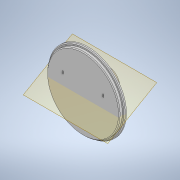
# Autodesk Inventor part: V4Lid
Saved by Autodesk Inventor 2021 (Build 250183000, 183)
## iProperties
Created: 2022-01-21
Part Number: V4Lid
Material: Generic
Document SubType Name: Sheet Metal
Designer: Unit-005
Density: 1 g/cm^3
Sheet Metal Rule: Default
Appearance: Default
Author: Unit-005
Autodesk Inventor part; units mm, degrees
ref_plane "YZ Plane" through (0, 0, 0) normal (1, 0, 0) x (0, 1, 0)
ref_plane "XY Plane" through (0, 0, 0) normal (0, 0, 1) x (1, 0, 0)
sketch "Sketch1" plane through (0, 0, 0) normal (0, 0, 1) x (1, 0, 0)
  circle A0 centre (0, 0) radius 19
  dimension "d0" = 38
  constraints: 1 centre point, 1 coincident
  measures "d0" diameter of A0
extrude "Extrusion1" add sketch "Sketch1" along normal blind 1
sketch "Sketch2" plane through (0, 0, 1) normal (0, 0, 1) x (1, 0, 0)
  circle A0 centre (0, 0) radius 17.95
  dimension "d3" = 35.9
  constraints: 1 centre point, 1 coincident
  measures "d3" diameter of A0
extrude "Extrusion2" add sketch "Sketch2" along normal blind 1.5
chamfer "Chamfer1" distance 0.4 angle 45 1 edges at (-17.95, 0, 2.5)
chamfer "Chamfer2" distance 0.4 angle 45 1 edges at (-19, 0, 1)
sketch "Sketch3" plane through (0, 0, 0) normal (0, 0, -1) x (-1, 0, 0)
  circle A0 centre (0, 0) radius 2
  dimension "d12" = 4
  constraints: 1 centre point, 1 coincident
  measures "d12" diameter of A0
extrude "Extrusion3" add sketch "Sketch3" along normal blind 10 draft 20
fillet "Fillet1" radius 5 1 edges at (2, 0, 0)
ref_plane "Work Plane1" through (0, 0, 0) normal (0, 0.8660254, 0.5) x (1, 0, 0)
sketch "Sketch4" plane through (0, 0, 0) normal (0, 0.8660254, 0.5) x (1, 0, 0)
  ellipse E0 centre (0, 0) end of major axis (19, 0) minor radius 9.5 projected
  ellipse E1 centre (0, 0) end of major axis (9.1407, 0) minor radius 4.5704 projected
  line L0 (-26.6, 0) -> (26.6, 0) projected
  circle A0 centre (10, 0) radius 0.375
  ellipse E2 centre (0, 0) end of major axis (9.1407, 0) minor radius 4.5704 projected
  dimension "d17" = 0.75
  dimension "d18" = 10
  constraints: 1 centre point, 1 point on line
  measures "d17" diameter of A0
  measures "d18" distance of E2.centre A0.centre
extrude "Extrusion4" cut sketch "Sketch4" along normal through all contours A0 L0 | L0 A0
mirror "Mirror1" about plane through (0, 0, 0) normal (1, 0, 0) of "Extrusion4"
equation "\"BendRadius\" = Thickness"
equation "\"BendReliefWidth\" = Thickness"
equation "\"BendReliefDepth\" = 0.5 * Thickness"
equation "\"CornerReliefSize\" = 4 * Thickness"
equation "\"MinimumRemnant\" = 2 * Thickness"
equation "\"TransitionRadius\" = BendRadius"
equation "\"JacobiRadiusSize\" = BendRadius"
equation "\"GapSize\" = Thickness"
equation "\"Thickness\" = 3.048"
body "Solid1"
